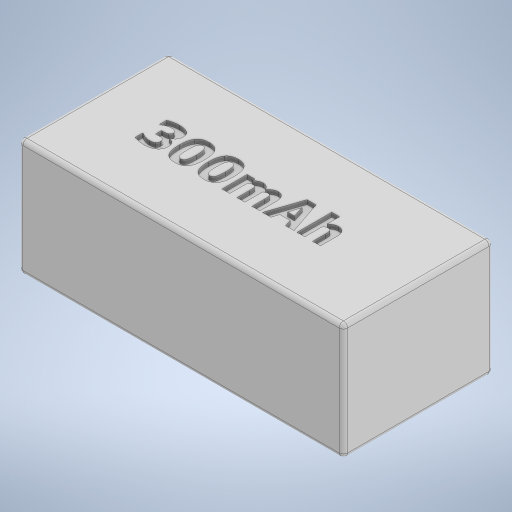
# Autodesk Inventor part: lipo-300
Saved by Autodesk Inventor 2023.5 (Build 275446000, 446)
## iProperties
Created: 2025-03-17
Part Number: lipo-300
Material: Ogólny
Document SubType Name: Modeling
Designer: kamil
Density: 1 g/cm^3
Appearance: Domyślna
Author: kamil
Autodesk Inventor part; units mm, degrees
ref_plane "YZ Plane" through (0, 0, 0) normal (1, 0, 0) x (0, 1, 0)
ref_plane "XZ Plane" through (0, 0, 0) normal (0, 1, 0) x (-1, 0, 0)
ref_plane "XY Plane" through (0, 0, 0) normal (0, 0, 1) x (1, 0, 0)
sketch "Szkic1" plane through (0, 0, 0) normal (0, 1, 0) x (-1, 0, 0)
  line L0 (0, 0) -> (-39, 0)
  line L1 (-39, 0) -> (-39, -18)
  line L2 (-39, -18) -> (0, -18)
  line L3 (0, -18) -> (0, 0)
  dimension "d0" = 39
  dimension "d1" = 18
  constraints: 8 end point, 2 parallel, 1 horizontal, 1 perpendicular
  measures "d0" distance of L2.end L1.end
  measures "d1" distance of L1.end L0.end
extrude "Wyciągnięcie proste1" add sketch "Szkic1" along normal blind 14
sketch "Szkic2" plane through (0, 14, 0) normal (0, 1, 0) x (1, 0, 0)
  line L0 (6.6151, 11.1072) -> (32.7116, 11.1072) construction
  line L1 (32.7116, 11.1072) -> (32.7116, 4.3277) construction
  line L2 (32.7116, 4.3277) -> (6.6151, 4.3277) construction
  line L3 (6.6151, 4.3277) -> (6.6151, 11.1072) construction
  spline S0 degree 2 poles (9.8598, 8.1412) (9.8598, 7.8462) (9.6426, 7.3633) (9.4319, 7.1947) knots 0 0 0 1 2 2 2
  spline S1 degree 2 poles (9.4319, 7.1947) (9.2212, 7.0261) (8.6475, 6.8446) (8.2358, 6.8446) knots 0 0 0 1 2 2 2
  spline S2 degree 2 poles (8.2358, 6.8446) (7.769, 6.8446) (7.1013, 7.0002) (6.8906, 7.0975) knots 0 0 0 1 2 2 2
  line L4 (6.8906, 7.0975) -> (6.8906, 7.9662)
  line L5 (6.8906, 7.9662) -> (6.9878, 7.9662)
  spline S3 degree 2 poles (6.9878, 7.9662) (7.2083, 7.8268) (7.8014, 7.6193) (8.0478, 7.6193) knots 0 0 0 1 2 2 2
  spline S4 degree 2 poles (8.0478, 7.6193) (8.1937, 7.6193) (8.534, 7.6712) (8.6507, 7.7555) knots 0 0 0 1 2 2 2
  spline S5 degree 2 poles (8.6507, 7.7555) (8.7415, 7.8236) (8.8517, 8.0213) (8.8517, 8.1996) knots 0 0 0 1 2 2 2
  spline S6 degree 2 poles (8.8517, 8.1996) (8.8517, 8.3778) (8.6961, 8.5691) (8.5664, 8.6145) knots 0 0 0 1 2 2 2
  spline S7 degree 2 poles (8.5664, 8.6145) (8.4368, 8.6599) (8.077, 8.6696) (7.9376, 8.6696) knots 0 0 0 1 2 2 2
  line L6 (7.9376, 8.6696) -> (7.7658, 8.6696)
  line L7 (7.7658, 8.6696) -> (7.7658, 9.373)
  line L8 (7.7658, 9.373) -> (7.9246, 9.373)
  spline S8 degree 2 poles (7.9246, 9.373) (8.1061, 9.373) (8.4141, 9.4054) (8.5211, 9.454) knots 0 0 0 1 2 2 2
  spline S9 degree 2 poles (8.5211, 9.454) (8.628, 9.5059) (8.748, 9.6874) (8.748, 9.843) knots 0 0 0 1 2 2 2
  spline S10 degree 2 poles (8.748, 9.843) (8.748, 9.9662) (8.6345, 10.1185) (8.5535, 10.1607) knots 0 0 0 1 2 2 2
  spline S11 degree 2 poles (8.5535, 10.1607) (8.4562, 10.2093) (8.1969, 10.2417) (8.1061, 10.2417) knots 0 0 0 1 2 2 2
  spline S12 degree 2 poles (8.1061, 10.2417) (7.9603, 10.2417) (7.6523, 10.1736) (7.5097, 10.1185) knots 0 0 0 1 2 2 2
  spline S13 degree 2 poles (7.5097, 10.1185) (7.3963, 10.0764) (7.1499, 9.9402) (7.0916, 9.9046) knots 0 0 0 1 2 2 2
  line L9 (7.0916, 9.9046) -> (7.0073, 9.9046)
  line L10 (7.0073, 9.9046) -> (7.0073, 10.7603)
  spline S14 degree 2 poles (7.0073, 10.7603) (7.2147, 10.8479) (7.9149, 11.0132) (8.2812, 11.0132) knots 0 0 0 1 2 2 2
  spline S15 degree 2 poles (8.2812, 11.0132) (8.6378, 11.0132) (9.1629, 10.89) (9.3476, 10.7701) knots 0 0 0 1 2 2 2
  spline S16 degree 2 poles (9.3476, 10.7701) (9.5519, 10.6437) (9.7561, 10.2547) (9.7561, 10.0116) knots 0 0 0 1 2 2 2
  spline S17 degree 2 poles (9.7561, 10.0116) (9.7561, 9.668) (9.3606, 9.1558) (9.0365, 9.0813) knots 0 0 0 1 2 2 2
  line L11 (9.0365, 9.0813) -> (9.0365, 9.0424)
  spline S18 degree 2 poles (9.0365, 9.0424) (9.1791, 9.0229) (9.4514, 8.9192) (9.581, 8.8025) knots 0 0 0 1 2 2 2
  spline S19 degree 2 poles (9.581, 8.8025) (9.701, 8.6988) (9.8598, 8.3681) (9.8598, 8.1412) knots 0 0 0 1 2 2 2
  spline S20 degree 2 poles (13.4125, 8.9289) (13.4125, 8.4103) (13.2472, 7.6323) (13.0624, 7.3697) knots 0 0 0 1 2 2 2
  spline S21 degree 2 poles (13.0624, 7.3697) (12.8809, 7.1104) (12.2942, 6.8446) (11.8728, 6.8446) knots 0 0 0 1 2 2 2
  spline S22 degree 2 poles (11.8728, 6.8446) (11.4481, 6.8446) (10.8647, 7.1104) (10.6799, 7.3762) knots 0 0 0 1 2 2 2
  spline S23 degree 2 poles (10.6799, 7.3762) (10.4951, 7.6388) (10.3298, 8.4103) (10.3298, 8.9289) knots 0 0 0 1 2 2 2
  spline S24 degree 2 poles (10.3298, 8.9289) (10.3298, 9.4605) (10.4951, 10.2125) (10.6831, 10.4848) knots 0 0 0 1 2 2 2
  spline S25 degree 2 poles (10.6831, 10.4848) (10.8711, 10.7506) (11.4643, 11.0099) (11.8728, 11.0099) knots 0 0 0 1 2 2 2
  spline S26 degree 2 poles (11.8728, 11.0099) (12.3039, 11.0099) (12.8809, 10.7377) (13.0656, 10.4686) knots 0 0 0 1 2 2 2
  spline S27 degree 2 poles (13.0656, 10.4686) (13.2472, 10.206) (13.4125, 9.4313) (13.4125, 8.9289) knots 0 0 0 1 2 2 2
  spline S28 degree 2 poles (12.4044, 8.9289) (12.4044, 9.6712) (12.1613, 10.2709) (11.8728, 10.2709) knots 0 0 0 1 2 2 2
  spline S29 degree 2 poles (11.8728, 10.2709) (11.5843, 10.2709) (11.3379, 9.6712) (11.3379, 8.9257) knots 0 0 0 1 2 2 2
  spline S30 degree 2 poles (11.3379, 8.9257) (11.3379, 8.1931) (11.5843, 7.5837) (11.8728, 7.5837) knots 0 0 0 1 2 2 2
  spline S31 degree 2 poles (11.8728, 7.5837) (12.158, 7.5837) (12.4044, 8.1931) (12.4044, 8.9289) knots 0 0 0 1 2 2 2
  spline S32 degree 2 poles (16.9165, 8.9289) (16.9165, 8.4103) (16.7512, 7.6323) (16.5664, 7.3697) knots 0 0 0 1 2 2 2
  spline S33 degree 2 poles (16.5664, 7.3697) (16.3849, 7.1104) (15.7982, 6.8446) (15.3768, 6.8446) knots 0 0 0 1 2 2 2
  spline S34 degree 2 poles (15.3768, 6.8446) (14.9522, 6.8446) (14.3687, 7.1104) (14.1839, 7.3762) knots 0 0 0 1 2 2 2
  spline S35 degree 2 poles (14.1839, 7.3762) (13.9992, 7.6388) (13.8339, 8.4103) (13.8339, 8.9289) knots 0 0 0 1 2 2 2
  spline S36 degree 2 poles (13.8339, 8.9289) (13.8339, 9.4605) (13.9992, 10.2125) (14.1872, 10.4848) knots 0 0 0 1 2 2 2
  spline S37 degree 2 poles (14.1872, 10.4848) (14.3752, 10.7506) (14.9684, 11.0099) (15.3768, 11.0099) knots 0 0 0 1 2 2 2
  spline S38 degree 2 poles (15.3768, 11.0099) (15.8079, 11.0099) (16.3849, 10.7377) (16.5697, 10.4686) knots 0 0 0 1 2 2 2
  spline S39 degree 2 poles (16.5697, 10.4686) (16.7512, 10.206) (16.9165, 9.4313) (16.9165, 8.9289) knots 0 0 0 1 2 2 2
  spline S40 degree 2 poles (15.9084, 8.9289) (15.9084, 9.6712) (15.6653, 10.2709) (15.3768, 10.2709) knots 0 0 0 1 2 2 2
  spline S41 degree 2 poles (15.3768, 10.2709) (15.0883, 10.2709) (14.842, 9.6712) (14.842, 8.9257) knots 0 0 0 1 2 2 2
  spline S42 degree 2 poles (14.842, 8.9257) (14.842, 8.1931) (15.0883, 7.5837) (15.3768, 7.5837) knots 0 0 0 1 2 2 2
  spline S43 degree 2 poles (15.3768, 7.5837) (15.6621, 7.5837) (15.9084, 8.1931) (15.9084, 8.9289) knots 0 0 0 1 2 2 2
  line L12 (21.0883, 6.9289) -> (21.0883, 8.4362)
  spline S44 degree 2 poles (21.0883, 8.4362) (21.0883, 8.6599) (21.0721, 8.9646) (21.0332, 9.0618) knots 0 0 0 1 2 2 2
  spline S45 degree 2 poles (21.0332, 9.0618) (20.9911, 9.159) (20.8225, 9.2466) (20.6702, 9.2466) knots 0 0 0 1 2 2 2
  spline S46 degree 2 poles (20.6702, 9.2466) (20.5632, 9.2466) (20.3557, 9.1526) (20.2326, 9.065) knots 0 0 0 1 2 2 2
  line L13 (20.2326, 9.065) -> (20.2326, 6.9289)
  line L14 (20.2326, 6.9289) -> (19.2861, 6.9289)
  line L15 (19.2861, 6.9289) -> (19.2861, 8.4362)
  spline S47 degree 2 poles (19.2861, 8.4362) (19.2861, 8.6566) (19.2666, 8.9646) (19.2277, 9.0618) knots 0 0 0 1 2 2 2
  spline S48 degree 2 poles (19.2277, 9.0618) (19.1856, 9.159) (19.017, 9.2466) (18.8647, 9.2466) knots 0 0 0 1 2 2 2
  spline S49 degree 2 poles (18.8647, 9.2466) (18.7512, 9.2466) (18.5275, 9.1396) (18.4238, 9.065) knots 0 0 0 1 2 2 2
  line L16 (18.4238, 9.065) -> (18.4238, 6.9289)
  line L17 (18.4238, 6.9289) -> (17.4838, 6.9289)
  line L18 (17.4838, 6.9289) -> (17.4838, 9.9467)
  line L19 (17.4838, 9.9467) -> (18.4238, 9.9467)
  line L20 (18.4238, 9.9467) -> (18.4238, 9.6129)
  spline S50 degree 2 poles (18.4238, 9.6129) (18.654, 9.8073) (19.0656, 10.0278) (19.3217, 10.0278) knots 0 0 0 1 2 2 2
  spline S51 degree 2 poles (19.3217, 10.0278) (19.5972, 10.0278) (20.0186, 9.7652) (20.1288, 9.5026) knots 0 0 0 1 2 2 2
  spline S52 degree 2 poles (20.1288, 9.5026) (20.3979, 9.7555) (20.8776, 10.0278) (21.124, 10.0278) knots 0 0 0 1 2 2 2
  spline S53 degree 2 poles (21.124, 10.0278) (21.3347, 10.0278) (21.6685, 9.8949) (21.782, 9.7587) knots 0 0 0 1 2 2 2
  spline S54 degree 2 poles (21.782, 9.7587) (21.9084, 9.6129) (22.0348, 9.2142) (22.0348, 8.8932) knots 0 0 0 1 2 2 2
  line L21 (22.0348, 8.8932) -> (22.0348, 6.9289)
  line L22 (22.0348, 6.9289) -> (21.0883, 6.9289)
  line L23 (22.3557, 6.9289) -> (23.7074, 10.9289)
  line L24 (23.7074, 10.9289) -> (24.8031, 10.9289)
  line L25 (24.8031, 10.9289) -> (26.1548, 6.9289)
  line L26 (26.1548, 6.9289) -> (25.1207, 6.9289)
  line L27 (25.1207, 6.9289) -> (24.8711, 7.7458)
  line L28 (24.8711, 7.7458) -> (23.6134, 7.7458)
  line L29 (23.6134, 7.7458) -> (23.3606, 6.9289)
  line L30 (23.3606, 6.9289) -> (22.3557, 6.9289)
  line L31 (24.6507, 8.4719) -> (24.2423, 9.7944)
  line L32 (24.2423, 9.7944) -> (23.8306, 8.4719)
  line L33 (23.8306, 8.4719) -> (24.6507, 8.4719)
  line L34 (29.3217, 6.9289) -> (28.3752, 6.9289)
  line L35 (28.3752, 6.9289) -> (28.3752, 8.4232)
  spline S55 degree 2 poles (28.3752, 8.4232) (28.3752, 8.608) (28.346, 8.971) (28.3071, 9.0553) knots 0 0 0 1 2 2 2
  spline S56 degree 2 poles (28.3071, 9.0553) (28.2585, 9.159) (28.077, 9.2466) (27.9214, 9.2466) knots 0 0 0 1 2 2 2
  spline S57 degree 2 poles (27.9214, 9.2466) (27.8079, 9.2466) (27.5713, 9.159) (27.4384, 9.065) knots 0 0 0 1 2 2 2
  line L36 (27.4384, 9.065) -> (27.4384, 6.9289)
  line L37 (27.4384, 6.9289) -> (26.4984, 6.9289)
  line L38 (26.4984, 6.9289) -> (26.4984, 11.1072)
  line L39 (26.4984, 11.1072) -> (27.4384, 11.1072)
  line L40 (27.4384, 11.1072) -> (27.4384, 9.6129)
  spline S58 degree 2 poles (27.4384, 9.6129) (27.6685, 9.8073) (28.1061, 10.0278) (28.372, 10.0278) knots 0 0 0 1 2 2 2
  spline S59 degree 2 poles (28.372, 10.0278) (28.8322, 10.0278) (29.3217, 9.4443) (29.3217, 8.8932) knots 0 0 0 1 2 2 2
  line L41 (29.3217, 8.8932) -> (29.3217, 6.9289)
  point P0 (0, 0)
  constraints: 2 other
extrude "Wyciągnięcie proste2" cut sketch "Szkic2" against normal blind 0.5
fillet "Zaokrąglenie1" radius 0.5 12 edges at (19.5, 14, 0) (39, 7, 0) (39, 14, -9) (39, 7, -18) (0, 7, -18) (19.5, 14, -18) (0, 14, -9) (0, 7, 0) (0, 0, -9) (19.5, 0, -18) (19.5, 0, 0) (39, 0, -9)
